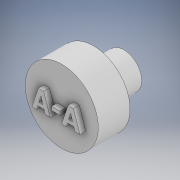
# Autodesk Inventor part: IPC A-A key
Saved by Autodesk Inventor 2022 (Build 260153000, 153)
## iProperties
Created: 2022-01-01
Part Number: IPC A-A key
Material: Generic
Document SubType Name: Modeling
Designer: solor
Density: 1 g/cm^3
Appearance: Default
Author: solor
Autodesk Inventor part; units mm, degrees
ref_plane "YZ Plane" through (0, 0, 0) normal (1, 0, 0) x (0, 1, 0)
ref_plane "XZ Plane" through (0, 0, 0) normal (0, 1, 0) x (-1, 0, 0)
ref_plane "XY Plane" through (0, 0, 0) normal (0, 0, 1) x (1, 0, 0)
sketch "Sketch1" plane through (0, 0, 0) normal (0, 0, 1) x (1, 0, 0)
  circle A0 centre (0, 0) radius 6.22 construction
  circle A1 centre (0, 0) radius 2.8
  line L0 (-0.675, 0.675) -> (-0.675, 2.025)
  line L1 (-0.675, 2.025) -> (0.675, 2.025)
  line L2 (0.675, 2.025) -> (0.675, 0.675)
  line L3 (0.675, 0.675) -> (2.025, 0.675)
  line L4 (2.025, 0.675) -> (2.025, -0.675)
  line L5 (2.025, -0.675) -> (0.675, -0.675)
  line L6 (0.675, -0.675) -> (0.675, -2.025)
  line L7 (0.675, -2.025) -> (-0.675, -2.025)
  line L8 (-0.675, -2.025) -> (-0.675, -0.675)
  line L9 (-0.675, -0.675) -> (-2.025, -0.675)
  line L10 (-2.025, -0.675) -> (-2.025, 0.675)
  line L11 (-2.025, 0.675) -> (-0.675, 0.675)
  circle A2 centre (0, 0) radius 5.75
  point P0 (-6.07, -6.1)
  dimension "d0" = 12.44
  dimension "d1" = 0.47
  constraints: 24 end point, 3 centre point, 1 coincident
  measures "d0" diameter of A0
  measures "d1" radial gap between concentric circles of A0 A2
extrude "Extrusion1" add sketch "Sketch1" along normal blind 5 contours A1 | L0 L1 L2 L3 L4 L5 L6 L7 L8 L9 L10 L11 | A2
extrude "Extrusion2" add sketch "Sketch1" against normal blind 4.8 contours A1
sketch "Sketch2" plane through (0, 0, 5) normal (0, 0, 1) x (1, 0, 0)
  point P0 (0, 0)
sketch "Sketch3" plane through (0, 0, 5) normal (0, 0, 1) x (1, 0, 0)
  line L0 (-3.7906, 1.533) -> (3.7906, 1.533) construction
  line L1 (3.7906, 1.533) -> (3.7906, -1.533) construction
  line L2 (3.7906, -1.533) -> (-3.7906, -1.533) construction
  line L3 (-3.7906, -1.533) -> (-3.7906, 1.533) construction
  line L4 (-3.803, -1.517) -> (-2.7723, 1.533)
  line L5 (-2.7723, 1.533) -> (-1.9369, 1.533)
  line L6 (-1.9369, 1.533) -> (-0.9062, -1.517)
  line L7 (-0.9062, -1.517) -> (-1.6947, -1.517)
  line L8 (-1.6947, -1.517) -> (-1.885, -0.8941)
  line L9 (-1.885, -0.8941) -> (-2.844, -0.8941)
  line L10 (-2.844, -0.8941) -> (-3.0368, -1.517)
  line L11 (-3.0368, -1.517) -> (-3.803, -1.517)
  line L12 (-2.0531, -0.3405) -> (-2.3645, 0.6679)
  line L13 (-2.3645, 0.6679) -> (-2.6784, -0.3405)
  line L14 (-2.6784, -0.3405) -> (-2.0531, -0.3405)
  line L15 (0.6633, -0.4542) -> (-0.6937, -0.4542)
  line L16 (-0.6937, -0.4542) -> (-0.6937, 0.1143)
  line L17 (-0.6937, 0.1143) -> (0.6633, 0.1143)
  line L18 (0.6633, 0.1143) -> (0.6633, -0.4542)
  line L19 (0.8783, -1.517) -> (1.909, 1.533)
  line L20 (1.909, 1.533) -> (2.7444, 1.533)
  line L21 (2.7444, 1.533) -> (3.7751, -1.517)
  line L22 (3.7751, -1.517) -> (2.9866, -1.517)
  line L23 (2.9866, -1.517) -> (2.7963, -0.8941)
  line L24 (2.7963, -0.8941) -> (1.8373, -0.8941)
  line L25 (1.8373, -0.8941) -> (1.6445, -1.517)
  line L26 (1.6445, -1.517) -> (0.8783, -1.517)
  line L27 (2.6282, -0.3405) -> (2.3168, 0.6679)
  line L28 (2.3168, 0.6679) -> (2.0029, -0.3405)
  line L29 (2.0029, -0.3405) -> (2.6282, -0.3405)
  point P0 (0, -1.533)
  point P1 (3.7906, 0)
  point P2 (0, 0)
  point P3 (0, 0)
  constraints: 2 midpoint, 2 other
extrude "Extrusion6" add sketch "Sketch3" along normal blind 0.9
body "Solid1"
